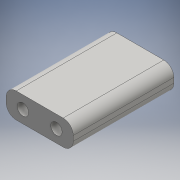
# Autodesk Inventor part: b1
Saved by Autodesk Inventor 2016 (Build 200138000, 138)
## iProperties
Created: 2016-09-21
Part Number: b1
Material: Generic
Document SubType Name: Modeling
Designer: Jakub
Density: 1 g/cm^3
Appearance: Default
Author: Jakub
Autodesk Inventor part; units mm, degrees
ref_plane "YZ Plane" through (0, 0, 0) normal (1, 0, 0) x (0, 1, 0)
ref_plane "XZ Plane" through (0, 0, 0) normal (0, 1, 0) x (-1, 0, 0)
ref_plane "XY Plane" through (0, 0, 0) normal (0, 0, 1) x (1, 0, 0)
sketch "Sketch1" plane through (0, 0, 0) normal (0, 1, 0) x (-1, 0, 0)
  line L0 (10, 3.75) -> (-10, 3.75)
  line L1 (-10, 3.75) -> (-10, -3.75)
  line L2 (-10, -3.75) -> (10, -3.75)
  line L3 (10, -3.75) -> (10, 3.75)
  line L4 (10, 3.75) -> (-10, -3.75) construction
  line L5 (-10, 3.75) -> (10, -3.75) construction
  circle A0 centre (5, 0) radius 1.7
  circle A1 centre (-5, 0) radius 1.7
  point P0 (0, 0)
  dimension "d0" = 20
  dimension "d1" = 7.5
  dimension "d2" = 3.4
  dimension "d3" = 3.4
  dimension "d4" = 5
  dimension "d5" = 5
  constraints: 12 end point, 2 centre point, 2 midpoint, 2 parallel, 1 horizontal, 1 perpendicular
  measures "d0" distance of L2.end L1.end
  measures "d1" distance of L1.end L0.end
  measures "d2" diameter of A0
  measures "d3" diameter of A1
  measures "d4" distance of point (0, 0) A0.centre
  measures "d5" distance of point (0, 0) A1.centre
extrude "Extrusion1" add sketch "Sketch1" along normal blind 30
fillet "Fillet1" radius 3 4 edges at (10, 15, 3.75) (10, 15, -3.75) (-10, 15, -3.75) (-10, 15, 3.75)
body "Solid1"
